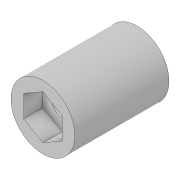
# Autodesk Inventor part: post
Saved by Autodesk Inventor 2019 (Build 230136000, 136)
## iProperties
Created: 2021-03-05
Part Number: post
Material: Generic
Document SubType Name: Modeling
Designer: LuoYi
Density: 1 g/cm^3
Appearance: Default
Author: LuoYi
Autodesk Inventor part; units mm, degrees
ref_plane "YZ Plane" through (0, 0, 0) normal (1, 0, 0) x (0, 1, 0)
ref_plane "XZ Plane" through (0, 0, 0) normal (0, 1, 0) x (-1, 0, 0)
ref_plane "XY Plane" through (0, 0, 0) normal (0, 0, 1) x (1, 0, 0)
sketch "Sketch1" plane through (0, 0, 0) normal (0, 0, 1) x (1, 0, 0)
  circle A0 centre (0, 0) radius 5
  dimension "d0" = 10
  constraints: 1 centre point, 1 coincident
  measures "d0" diameter of A0
extrude "Extrusion1" add sketch "Sketch1" along normal blind 14.75
sketch "Sketch2" plane through (0, 0, 14.75) normal (0, 0, 1) x (1, 0, 0)
  circle A0 centre (0, 0) radius 1.6
  dimension "d3" = 3.2
  constraints: 1 centre point, 1 coincident
  measures "d3" diameter of A0
extrude "Extrusion2" cut sketch "Sketch2" against normal blind 14.75
sketch "Sketch3" plane through (0, 0, 14.75) normal (0, 0, 1) x (1, 0, 0)
  line L0 (0, 3.4641) -> (3, 1.7321)
  line L1 (3, 1.7321) -> (3, -1.7321)
  line L2 (3, -1.7321) -> (0, -3.4641)
  line L3 (0, -3.4641) -> (-3, -1.7321)
  line L4 (-3, -1.7321) -> (-3, 1.7321)
  line L5 (-3, 1.7321) -> (0, 3.4641)
  point P0 (0, 0)
  point P1 (0, 0)
  dimension "d6" = 6
  constraints: 12 end point, 1 coincident, 1 vertical, 13 other
  measures "d6" distance between parallel lines of L4 L1
extrude "Extrusion3" cut sketch "Sketch3" against normal blind 3
sketch "Sketch4" plane through (0, 0, 0) normal (0, 0, -1) x (-1, 0, 0)
  circle A0 centre (0, 0) radius 1.6 projected
  line L0 (0, 3.4641) -> (-3, 1.7321) projected
  line L1 (3, 1.7321) -> (0, 3.4641) projected
  line L2 (3, -1.7321) -> (3, 1.7321) projected
  line L3 (0, -3.4641) -> (3, -1.7321) projected
  line L4 (-3, -1.7321) -> (0, -3.4641) projected
  line L5 (-3, 1.7321) -> (-3, -1.7321) projected
extrude "Extrusion4" cut sketch "Sketch4" against normal blind 3
body "Solid1"
